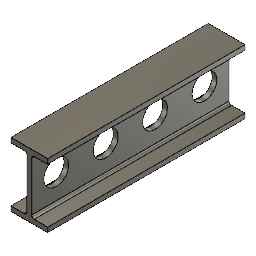
I-Beam (Autodesk Fusion 360 design; units mm, degrees)
Autodesk Fusion 360 part; units mm, degrees
sketch "Sketch1" plane through (0, 0, 0) normal (0, 0, 1) x (1, 0, 0)
  line L0 (0, 0) -> (97.8805, 0) construction
  line L1 (0.5, 0) -> (0.5, 5)
  arc A0 (1, 5.5) -> (0.5, 5) centre (1, 5) ccw
  line L2 (1, 5.5) -> (3.75, 5.5)
  line L3 (3.75, 5.5) -> (3.75, 6.5)
  line L4 (3.75, 6.5) -> (0, 6.5)
  line L5 (0, 0) -> (0, 6.5) construction
  line L6 (-3.75, 6.5) -> (0, 6.5)
  line L7 (-3.75, 5.5) -> (-3.75, 6.5)
  line L8 (-1, 5.5) -> (-3.75, 5.5)
  arc A1 (-0.5, 5) -> (-1, 5.5) centre (-1, 5) ccw
  line L9 (-0.5, 0) -> (-0.5, 5)
  line L10 (-3.75, -6.5) -> (0, -6.5)
  line L11 (-3.75, -5.5) -> (-3.75, -6.5)
  line L12 (-1, -5.5) -> (-3.75, -5.5)
  arc A2 (-1, -5.5) -> (-0.5, -5) centre (-1, -5) ccw
  line L13 (-0.5, 0) -> (-0.5, -5)
  line L14 (0.5, 0) -> (0.5, -5)
  arc A3 (0.5, -5) -> (1, -5.5) centre (1, -5) ccw
  line L15 (1, -5.5) -> (3.75, -5.5)
  line L16 (3.75, -5.5) -> (3.75, -6.5)
  line L17 (3.75, -6.5) -> (0, -6.5)
  dimension "d1" = 0.5
  dimension "d2" = 0.5
  dimension "d3" = 1
  dimension "d4" = 5.5
  dimension "d5" = 3.25
  constraint coincident L0.start L5.start
  constraint horizontal L0
  constraint coincident L0 L1.start
  constraint perpendicular L0 L1
  constraint tangent L1 A0
  constraint perpendicular L1 L2
  constraint perpendicular L2 L3
  constraint perpendicular L3 L4
  constraint vertical L5
  constraint tangent A0 L2
  constraint symmetric L1.start L5 L9.start
  constraint symmetric L1.end L5 A1.start
  constraint symmetric A0.start L5 L8.start
  constraint symmetric A0 L5 A1
  constraint symmetric L2.end L5 L7.start
  constraint symmetric L3.end L5 L6.start
  constraint symmetric L4.end L5 L6.end
  constraint symmetric L0 L1.start L14.start
  constraint symmetric L0 L1.end L14.end
  constraint symmetric L0 A0.start A3.end
  constraint symmetric L0 A0 A3
  constraint symmetric L0 L2.end L15.end
  constraint symmetric L0 L3.end L16.end
  constraint symmetric L0 L4.end L10.end
  constraint symmetric L0 L6.start L10.start
  constraint symmetric L0 L7.start L11.start
  constraint symmetric L0 L8.start L12.start
  constraint symmetric L0 A1.start A2.end
  constraint symmetric L0 A1 A2
  constraint symmetric L0 L9.start L13.start
  measures "d1" radius of A0
  measures "d2" distance of L0.start L1
  measures "d3" distance of L2.end L3.end
  measures "d4" distance of L0 L2
  measures "d5" horizontal distance of L1.end L2.end
extrude "Extrude1" add sketch "Sketch1" along normal blind 40
sketch "Sketch2" plane through (0.5, 0, 0) normal (1, 0, 0) x (0, 0, -1)
  line L0 (0, -5) -> (0, 5)
  line L1 (0, 5) -> (-40, 5)
  line L2 (-40, 5) -> (-40, -5)
  line L3 (-40, -5) -> (0, -5)
  line L4 (0, 0) -> (-40, 0) construction
  circle A0 centre (-35, 0) radius 2.5
  circle A1 centre (-25, 0) radius 2.5
  circle A2 centre (-15, 0) radius 2.5
  circle A3 centre (-5, 0) radius 2.5
  point P0 (-5, 0)
  point P1 (-25, 0)
  point P2 (-35, 0)
  point P3 (-15, 0)
  dimension "d8" = 5
  dimension "d9" = 15
  dimension "d10" = 25
  dimension "d11" = 35
  dimension "d12" = 5
  dimension "d13" = 5
  dimension "d14" = 5
  dimension "d15" = 5
  constraint coincident L4.start origin
  constraint midpoint L2 L4.end
  constraint coincident P0 L4
  constraint coincident P1 L4
  constraint coincident P2 L4
  constraint coincident L4 P3
  constraint coincident P2 A0.centre
  constraint coincident P1 A1.centre
  constraint coincident P3 A2.centre
  constraint coincident P0 A3.centre
  measures "d8" distance of P2 L4.end
  measures "d9" distance of P1 L4.end
  measures "d10" distance of L4.end P3
  measures "d11" distance of P0 L4.end
  measures "d12" diameter of A0
  measures "d13" diameter of A1
  measures "d14" diameter of A2
  measures "d15" diameter of A3
extrude "Extrude2" cut sketch "Sketch2" against normal through all contours A0 | A1 | A2 | A3
